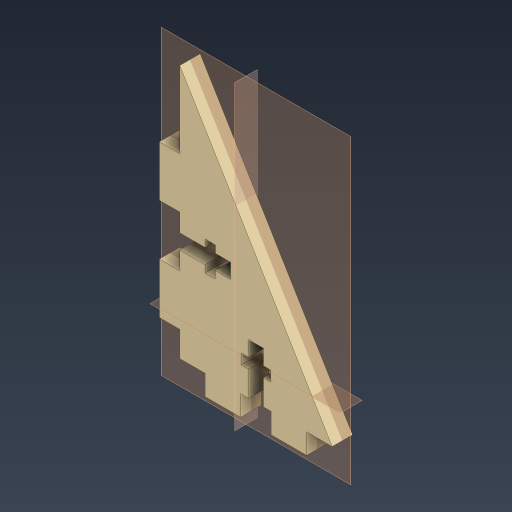
# Autodesk Inventor part: Рёбра_жёсткости
Saved by Autodesk Inventor 2023.2 (Build 272271030, 271C)
## iProperties
Created: 2025-12-29
Part Number: Рёбра_жёсткости
Material: Типовые
Document SubType Name: Modeling
Designer: Олег Коноваленко
Density: 1 g/cm^3
Appearance: Пшеничный
Author: Олег Коноваленко
Autodesk Inventor part; units mm, degrees
sketch "Эскиз1" plane through (0, 0, 0) normal (0, 0, 1) x (1, 0, 0)
  line L0 (-11.0294, 43.3824) -> (-11.0294, -6.6176)
  line L1 (-11.0294, -6.6176) -> (18.9706, -6.6176)
  line L2 (18.9706, -6.6176) -> (-11.0294, 43.3824)
  line L3 (-11.0294, -6.6176) -> (11.0294, 6.6176) construction
  line L4 (-6.0294, -6.6176) -> (0.9706, -6.6176)
  line L5 (0.9706, -6.6176) -> (0.9706, -10.6176)
  line L6 (0.9706, -10.6176) -> (-6.0294, -10.6176)
  line L7 (-6.0294, -10.6176) -> (-6.0294, -6.6176)
  line L8 (6.9706, -6.6176) -> (13.9706, -6.6176)
  line L9 (13.9706, -6.6176) -> (13.9706, -10.6176)
  line L10 (13.9706, -10.6176) -> (6.9706, -10.6176)
  line L11 (6.9706, -10.6176) -> (6.9706, -6.6176)
  line L12 (-11.0294, 28.3824) -> (-15.0294, 28.3824)
  line L13 (-15.0294, 28.3824) -> (-15.0294, 18.3824)
  line L14 (-15.0294, 18.3824) -> (-11.0294, 18.3824)
  line L15 (-11.0294, 18.3824) -> (-11.0294, 28.3824)
  line L16 (-11.0294, -1.6176) -> (-15.0294, -1.6176)
  line L17 (-15.0294, -1.6176) -> (-15.0294, 8.3824)
  line L18 (-15.0294, 8.3824) -> (-11.0294, 8.3824)
  line L19 (-11.0294, 8.3824) -> (-11.0294, -1.6176)
  point P0 (0, 0)
  point P1 (0, 0)
  point P2 (-11.0294, 8.3824)
  point P3 (0.9706, -6.6176)
  dimension "d0" = 30
  dimension "d1" = 50
  dimension "d2" = 10
  dimension "d3" = 15
  dimension "d4" = 4
  dimension "d5" = 5
  dimension "d6" = 5
  dimension "d7" = 7
  dimension "d8" = 5
  constraints: 40 end point, 8 parallel, 6 perpendicular, 5 equal length, 5 point on line, 4 horizontal, 1 coincident, 1 midpoint, 1 vertical
  measures "d0" distance of L0.end L1.end
  measures "d1" distance of L0.start L0.end
  measures "d2" distance of L12.end L13.end
  measures "d3" distance from line of L0.start L12
  measures "d4" distance of L13.end L14.end
  measures "d5" distance from line of L0.end L16
  measures "d6" distance from line of L0.end L7
  measures "d7" distance of L5.end L6.end
  measures "d8" distance from line of L1.end L9
extrude "Выдавливание1" add sketch "Эскиз1" along normal mid plane 4
sketch "Эскиз2" plane through (0, 0, 2) normal (0, 0, 1) x (1, 0, 0)
  line L0 (-11.0294, 18.3824) -> (-11.0294, 8.3824) projected
  line L1 (-11.0294, 14.8324) -> (-1.0294, 14.8324)
  line L2 (-1.0294, 14.8324) -> (-1.0294, 11.9324)
  line L3 (-1.0294, 11.9324) -> (-11.0294, 11.9324)
  line L4 (-11.0294, 11.9324) -> (-11.0294, 14.8324)
  line L5 (0.9706, -6.6176) -> (6.9706, -6.6176) projected
  line L6 (2.5206, -6.6176) -> (5.4206, -6.6176)
  line L7 (5.4206, -6.6176) -> (5.4206, 3.3824)
  line L8 (5.4206, 3.3824) -> (2.5206, 3.3824)
  line L9 (2.5206, 3.3824) -> (2.5206, -6.6176)
  line L10 (-6.0294, 16.2824) -> (-4.0294, 16.2824)
  line L11 (-4.0294, 16.2824) -> (-4.0294, 10.4824)
  line L12 (-4.0294, 10.4824) -> (-6.0294, 10.4824)
  line L13 (-6.0294, 10.4824) -> (-6.0294, 16.2824)
  line L14 (1.0706, 0.3824) -> (6.8706, 0.3824)
  line L15 (6.8706, 0.3824) -> (6.8706, -1.6176)
  line L16 (6.8706, -1.6176) -> (1.0706, -1.6176)
  line L17 (1.0706, -1.6176) -> (1.0706, 0.3824)
  line L18 (-11.0294, 13.3824) -> (-1.0294, 13.3824) construction
  line L19 (3.9706, 3.3824) -> (3.9706, -6.6176) construction
  point P0 (0, 0)
  point P1 (-4.0294, 13.3824)
  point P2 (3.9706, 0.3824)
  point P3 (-6.0294, 14.8324)
  point P4 (-11.0294, 11.9324)
  point P5 (-6.0294, 11.9324)
  point P6 (-4.0294, 11.9324)
  point P7 (-4.0294, 14.8324)
  point P8 (2.5206, -1.6176)
  point P9 (5.4206, -1.6176)
  point P10 (5.4206, 0.3824)
  point P11 (2.5206, 0.3824)
  dimension "d11" = 2.9
  dimension "d12" = 10
  dimension "d13" = 2
  dimension "d14" = 5.8
  dimension "d15" = 5
  dimension "d16" = 5
  constraints: 36 end point, 8 midpoint, 8 parallel, 8 perpendicular, 4 horizontal, 4 point on line, 1 vertical
  measures "d11" distance of L1.end L2.end
  measures "d12" distance of L2.end L3.end
  measures "d13" distance of L10.start L10.end
  measures "d14" distance of L10.end L11.end
  measures "d15" distance between parallel lines of L0 L13
  measures "d16" distance between parallel lines of L5 L16
extrude "Выдавливание2" cut sketch "Эскиз2" against normal up to next
